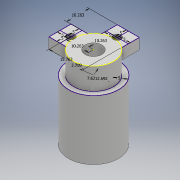
# Autodesk Inventor part: springHolder_final
Saved by Autodesk Inventor 2018 (Build 220112000, 112)
## iProperties
Created: 2017-11-09
Part Number: springHolder_final
Material: Generic
Document SubType Name: Modeling
Designer: Payal Jindal
Density: 1 g/cm^3
Appearance: Default
Author: Payal Jindal
Autodesk Inventor part; units mm, degrees
ref_plane "YZ Plane" through (0, 0, 0) normal (1, 0, 0) x (0, 1, 0)
ref_plane "XZ Plane" through (0, 0, 0) normal (0, 1, 0) x (-1, 0, 0)
ref_plane "XY Plane" through (0, 0, 0) normal (0, 0, 1) x (1, 0, 0)
sketch "Sketch1" plane through (0, 0, 0) normal (0, 0, 1) x (1, 0, 0)
  circle A0 centre (0, 0) radius 6.346
  circle A1 centre (0, 0) radius 11.346
  circle A2 centre (0, 0) radius 3.81
  circle A3 centre (0, 0) radius 9.0554
  dimension "d0" = 12.692
  dimension "d1" = 5
  dimension "d2" = 7.62
  dimension "d7" = 2.7094
  constraints: 4 centre point, 3 coincident
  measures "d0" diameter of A0
  measures "d1" radial gap between concentric circles of A1 A0
  measures "d2" diameter of A2
  measures "d7" radial gap between concentric circles of A0 A3
extrude "Extrusion1" add sketch "Sketch1" against normal blind 27.225 contours A1 | A3
extrude "Extrusion3" add sketch "Sketch1" along normal blind 10 contours A0 | A3
sketch "Sketch2" plane through (0, 0, 10) normal (0, 0, 1) x (1, 0, 0)
  line L0 (0.5, 10.2508) -> (5.5, 10.2508)
  line L1 (0.5, 10.2508) -> (-4.5, 10.2508)
  line L2 (0.5, 10.2508) -> (0.5, 15.2508)
  line L3 (-10.263, -0.0122) -> (-10.263, 4.9878)
  line L4 (-10.263, -0.0122) -> (-15.263, -0.0122)
  line L5 (-10.263, -0.0122) -> (-10.263, -5.0122)
  line L6 (-10.263, 4.9878) -> (-7.5579, 4.9878)
  circle A0 centre (0, 0) radius 9.0554 projected
  line L7 (-10.263, 4.9878) -> (-15.263, 4.9878)
  line L8 (-15.263, 4.9878) -> (-15.263, -0.0122)
  line L9 (-10.263, -5.0122) -> (-7.5417, -5.0122)
  line L10 (-10.263, -5.0122) -> (-15.263, -5.0122)
  line L11 (-15.263, -5.0122) -> (-15.263, -0.0122)
  line L12 (0.5, 15.2508) -> (5.5, 15.2508)
  line L13 (5.5, 15.2508) -> (5.5, 10.2508)
  line L14 (5.5, 10.2508) -> (5.5, 7.1937)
  line L15 (0.5, 15.2508) -> (-4.5, 15.2508)
  line L16 (-4.5, 15.2508) -> (-4.5, 10.2508)
  line L17 (-4.5, 7.8581) -> (-4.5, 10.2508)
  dimension "d10" = 10.263
  dimension "d11" = 10.263
  dimension "d12" = 5
  dimension "d13" = 5
  dimension "d14" = 5
  dimension "d15" = 5
  dimension "d16" = 5
  dimension "d17" = 5
  dimension "d18" = 15.763
  dimension "d19" = 10.263
  constraints: 36 end point, 8 horizontal, 4 perpendicular, 4 point on circle, 4 vertical, 2 coincident, 2 point on line, 1 collinear
  measures "d10" distance of point (0, 0) L0.start
  measures "d11" distance of point (0, 0) L3.start
  measures "d12" distance of L0.start L0.end
  measures "d13" distance of L0.start L1.end
  measures "d14" distance of L0.start L2.end
  measures "d15" distance of L3.start L3.end
  measures "d16" distance of L3.start L4.end
  measures "d17" distance of L3.start L5.end
  measures "d18" distance between parallel lines of L14 L5
  measures "d19" distance between parallel lines of L15 L7
extrude "Extrusion4" add sketch "Sketch2" against normal blind 5 contours L2 L12 L13 L0 | L0 L14 A0 L17 L1 | L1 L16 L15 L2 | A0 L9 L5 L3 L6 | L3 L4 L8 L7 | L10 L11 L4 L5
sketch "Sketch4" plane through (0, 0, 5) normal (0, 0, -1) x (-1, 0, 0)
  line L0 (-5.5, 15.2508) -> (4.5, 15.2508) projected
  line L1 (-0.5, 15.2508) -> (-0.5, 9.7508)
  line L2 (3.5, 7.4414) -> (-0.5, 5.132)
  line L3 (-0.5, 5.132) -> (-4.5, 7.4414)
  line L4 (-4.5, 7.4414) -> (-4.5, 12.0602)
  line L5 (-4.5, 12.0602) -> (-0.5, 14.3696)
  line L6 (-0.5, 14.3696) -> (3.5, 12.0602)
  line L7 (3.5, 12.0602) -> (3.5, 7.4414)
  point P0 (0, 0)
  point P1 (3.5, 9.7508)
  dimension "d22" = 5.5
  dimension "d23" = 8
  constraints: 14 end point, 2 midpoint, 2 vertical, 1 coincident, 13 other
  measures "d22" distance of L1.start L1.end
  measures "d23" distance between parallel lines of L3 L6
extrude "Extrusion5" cut sketch "Sketch4" along normal mid plane 5
sketch "Sketch5" plane through (0, 0, 5) normal (0, 0, -1) x (-1, 0, 0)
  line L0 (15.263, 4.9878) -> (15.263, -5.0122) projected
  line L1 (15.263, -0.0122) -> (9.763, -0.0122)
  line L2 (7.4536, -4.0122) -> (5.1442, -0.0122)
  line L3 (5.1442, -0.0122) -> (7.4536, 3.9878)
  line L4 (7.4536, 3.9878) -> (12.0724, 3.9878)
  line L5 (12.0724, 3.9878) -> (14.3818, -0.0122)
  line L6 (14.3818, -0.0122) -> (12.0724, -4.0122)
  line L7 (12.0724, -4.0122) -> (7.4536, -4.0122)
  line L8 (3.5, 12.0602) -> (3.5, 7.4414) projected
  point P0 (0, 0)
  dimension "d26" = 5.5
  constraints: 14 end point, 2 horizontal, 1 coincident, 1 midpoint, 1 perpendicular, 13 other
  measures "d26" distance of L1.start L1.end
extrude "Extrusion6" cut sketch "Sketch5" along normal mid plane 5
hole "Hole1" at (0.5, 10.2508, 10) at (-10.263, -0.0122, 10) direction (0, 0, -1) diameter 3.5 depth 6.25 tip angle 118
body "Solid1"
